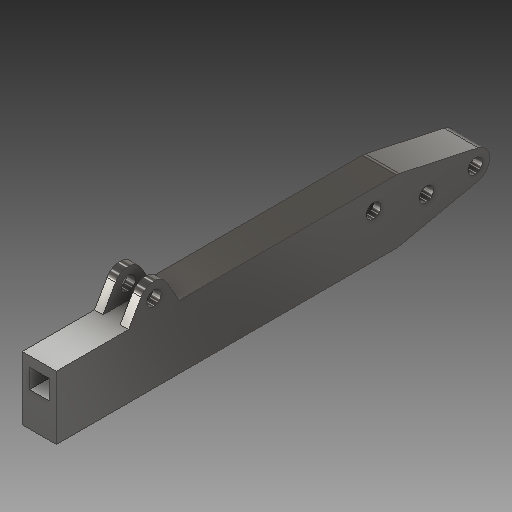
# Autodesk Inventor part: DipperSon
Saved by Autodesk Inventor 2019 (Build 230136000, 136)
## iProperties
Created: 2018-12-27
Part Number: DipperSon
Material: 钢，高强度，低合金
Document SubType Name: Modeling
Designer: JianQiao Hu
Density: 7.85 g/cm^3
Appearance: 钢 - 抛光
Author: JianQiao Hu
Autodesk Inventor part; units mm, degrees
note: some values were not read from the file. Chosen so that the rebuilt part matches the saved one: arc direction of "拉伸6".
ref_plane "YZ Plane" through (0, 0, 0) normal (1, 0, 0) x (0, 1, 0)
ref_plane "XZ Plane" through (0, 0, 0) normal (0, 1, 0) x (-1, 0, 0)
ref_plane "XY Plane" through (0, 0, 0) normal (0, 0, 1) x (1, 0, 0)
sketch "草图1" plane through (0, 0, 0) normal (0, 0, 1) x (1, 0, 0)
  line L0 (-35, 65) -> (35, 65)
  line L1 (35, 65) -> (35, -65)
  line L2 (35, -65) -> (-35, -65)
  line L3 (-35, -65) -> (-35, 65)
  line L4 (-35, 65) -> (35, -65) construction
  line L5 (35, 65) -> (-35, -65) construction
  point P0 (0, 0)
  dimension "d0" = 70
  dimension "d1" = 130
  constraints: 12 end point, 2 midpoint, 2 parallel, 1 horizontal, 1 perpendicular
  measures "d0" distance of L1.end L2.end
  measures "d1" distance of L0.end L1.end
extrude "拉伸1" add sketch "草图1" along normal blind 1000
sketch "草图2" plane through (-35, -65, 0) normal (-1, 0, 0) x (0, 0, 1)
  line L0 (0, 65) -> (300, 0)
  line L1 (0, 0) -> (1000, 0) projected
  line L2 (0, 130) -> (1000, 130) projected
  line L3 (300, 130) -> (0, 65)
  line L4 (300, 0) -> (300, 130)
  line L5 (0, 0) -> (0, 130) projected
  dimension "d4" = 300
  constraints: 6 end point, 2 point on line, 1 vertical
  measures "d4" distance between parallel lines of L5 L4
extrude "拉伸2" cut sketch "草图2" against normal through all contours L5 L2 L3 | L0 L1 L5
fillet "圆角1" radius 30 3 edges at (0, 0, 0) (0, 65, 300) (0, -65, 300)
sketch "草图3" plane through (-35, -65, 1000) normal (-1, 0, 0) x (0, 0, 1)
  arc A0 (-864.6783, 94.3197) -> (-864.6783, 35.6803) centre (-858.3257, 65) ccw projected
  circle A1 centre (-858.3257, 65) radius 15
  circle A2 centre (-758.3257, 65) radius 15
  point P0 (-1000, 65)
  dimension "d8" = 30
  dimension "d11" = 30
  dimension "d12" = 100
  constraints: 2 centre point, 1 coincident
  measures "d8" diameter of A1
  measures "d11" diameter of A2
  measures "d12" distance of A2.centre A1.centre
extrude "拉伸3" cut sketch "草图3" against normal through all
sketch "草图4" plane through (0, 0, 1000) normal (0, 0, 1) x (1, 0, 0)
  line L0 (-53.3891, 25) -> (64.6192, 25)
  line L1 (0, 81.4777) -> (0, 16.0102)
  line L2 (-20, 45) -> (20, 45)
  line L3 (20, 45) -> (20, 5)
  line L4 (20, 5) -> (-20, 5)
  line L5 (-20, 5) -> (-20, 45)
  line L6 (-20, 45) -> (20, 5) construction
  line L7 (20, 45) -> (-20, 5) construction
  line L8 (35, 65) -> (-35, 65) projected
  point P0 (0, 0)
  point P1 (0, 25)
  dimension "d13" = 40
  dimension "d14" = 40
  dimension "d15" = 40
  constraints: 16 end point, 2 horizontal, 2 midpoint, 2 parallel, 2 point on line, 1 perpendicular, 1 vertical
  measures "d13" distance between parallel lines of L8 L0
  measures "d14" distance of L2.start L2.end
  measures "d15" distance of L2.end L3.end
extrude "拉伸4" cut sketch "草图4" against normal blind 700
sketch "草图5" plane through (-20, 5, 1000) normal (1, 0, 0) x (0, 0, -1)
  line L0 (-16.4327, 20) -> (719.4245, 20)
  line L1 (696.7873, 60) -> (0, 60) projected
  circle A0 centre (650, 20) radius 15
  line L2 (0, -70) -> (0, 60) projected
  point P0 (1000, -5)
  dimension "d18" = 40
  dimension "d19" = 30
  dimension "d20" = 650
  constraints: 2 end point, 1 centre point, 1 horizontal, 1 point on line
  measures "d18" distance between parallel lines of L1 L0
  measures "d19" diameter of A0
  measures "d20" distance from line of L2 A0.centre
extrude "拉伸5" cut sketch "草图5" along normal mid plane 700
sketch "草图6" plane through (0, 0, 0) normal (1, 0, 0) x (0, 1, 0)
  circle A0 centre (95, 800) radius 15
  line L0 (65, 303.2127) -> (65, 1000) projected
  line L1 (-65, 1000) -> (65, 1000) projected
  line L2 (95.8043, 829.9892) -> (131.374, 829.9892) construction
  line L3 (109.6775, 773.8357) -> (183.0515, 773.8357) construction
  line L4 (65, 847.7741) -> (65, 745.182)
  circle A1 centre (95, 800) radius 30
  line L5 (110.3646, 825.7668) -> (65, 851.9581)
  line L6 (110.3646, 825.7668) -> (162.747, 825.7668) construction
  line L7 (65, 851.9581) -> (65, 745.182)
  line L8 (65, 303.2127) -> (65, 1000) projected
  line L9 (111.8573, 775.184) -> (65, 748.131)
  line L10 (111.8573, 775.184) -> (168.7185, 775.184) construction
  point P0 (0, 0)
  dimension "d23" = 30
  dimension "d25" = 30
  dimension "d26" = 200
  dimension "d29" = 60
  dimension "d30" = 150
  dimension "d31" = 150
  constraints: 16 end point, 4 horizontal, 3 point on line, 2 centre point, 2 point on circle, 1 coincident, 1 collinear, 1 equal length
  measures "d23" diameter of A0
  measures "d25" distance from line of L0 A0.centre
  measures "d26" distance from line of L1 A0.centre
  measures "d29" diameter of A1
  measures "d30" angle of L6 L5
  measures "d31" angle of L9 L10
extrude "拉伸6" add sketch "草图6" along normal mid plane 70
sketch "草图7" plane through (-35, 65, 1000) normal (0, 1, 0) x (1, 0, 0)
  line L0 (70, 148.0419) -> (0, 148.0419) projected
  line L1 (35, 148.0419) -> (35, 251.869)
  line L2 (0, 251.869) -> (70, 251.869) projected
  line L3 (0, 185) -> (0, 215) projected
  line L4 (0, 200) -> (70.1178, 200)
  line L5 (17.5589, 104.0655) -> (52.5589, 104.0655)
  line L6 (52.5589, 104.0655) -> (52.5589, 295.9345)
  line L7 (52.5589, 295.9345) -> (17.5589, 295.9345)
  line L8 (17.5589, 295.9345) -> (17.5589, 104.0655)
  line L9 (17.5589, 104.0655) -> (52.5589, 295.9345) construction
  line L10 (52.5589, 104.0655) -> (17.5589, 295.9345) construction
  point P0 (35, 1000)
  point P1 (35.0589, 200)
  dimension "d35" = 35
  constraints: 16 end point, 6 midpoint, 2 horizontal, 2 parallel, 1 perpendicular
  measures "d35" distance of L6.end L7.end
extrude "拉伸7" cut sketch "草图7" along normal blind 70
